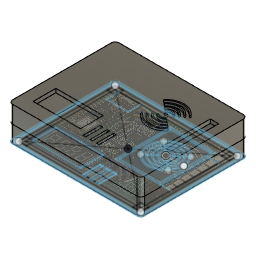
RFIDBox v2 (Autodesk Fusion 360 design; units mm, degrees)
Autodesk Fusion 360 part; units mm, degrees
note: some values were not read from the file. Chosen so that the rebuilt part matches the saved one: which bodies a step acts on; which face or edge a step refers to. Set by a fixed rule: which sketch regions a step uses.
sketch "Sketch1" plane through (0, 0, 0) normal (0, 0, 1) x (1, 0, 0)
  line L0 (47.5, -37.5) -> (-47.5, -37.5)
  line L1 (-47.5, -37.5) -> (-47.5, 37.5)
  line L2 (-47.5, 37.5) -> (47.5, 37.5)
  line L3 (47.5, 37.5) -> (47.5, -37.5)
  line L4 (47.5, -37.5) -> (-47.5, 37.5) construction
  line L5 (-47.5, -37.5) -> (47.5, 37.5) construction
  line L6 (45, -35) -> (-45, -35)
  line L7 (-45, -35) -> (-45, 35)
  line L8 (-45, 35) -> (45, 35)
  line L9 (45, 35) -> (45, -35)
  line L10 (45, -35) -> (-45, 35) construction
  line L11 (-45, -35) -> (45, 35) construction
  line L12 (-42.4055, -13.8661) -> (-5.5569, -13.8661)
  line L13 (-5.5569, -13.8661) -> (-5.5569, -31.5415)
  line L14 (-5.5569, -31.5415) -> (-42.4055, -31.5415)
  line L15 (-42.4055, -31.5415) -> (-42.4055, -13.8661)
  line L16 (38.4816, 25.6787) -> (45, 25.6787)
  line L17 (45, 25.6787) -> (45, -11.6193)
  line L18 (45, -11.6193) -> (38.4816, -11.6193)
  line L19 (38.4816, -11.6193) -> (38.4816, 25.6787)
  line L20 (2.0824, 31.0711) -> (36.6841, 31.0711)
  line L21 (36.6841, 31.0711) -> (36.6841, -11.6193)
  line L22 (36.6841, -11.6193) -> (2.0824, -11.6193)
  line L23 (2.0824, -11.6193) -> (2.0824, 31.0711)
  line L24 (-41.6565, 35) -> (-25, 35)
  line L25 (-25, 35) -> (-25, 25)
  line L26 (-25, 25) -> (-41.6565, 25)
  line L27 (-41.6565, 25) -> (-41.6565, 35)
  line L28 (0, -21.6553) -> (12.418, -21.6553)
  line L29 (12.418, -21.6553) -> (12.418, -35)
  line L30 (12.418, -35) -> (0, -35)
  line L31 (0, -35) -> (0, -21.6553)
  line L32 (-48.5, 41.5) -> (48.5, 41.5)
  line L33 (51.5, 38.5) -> (51.5, -38.5)
  line L34 (48.5, -41.5) -> (-48.5, -41.5)
  line L35 (-51.5, -38.5) -> (-51.5, 38.5)
  line L36 (-47.5, 39.5) -> (47.5, 39.5)
  line L37 (49.5, 37.5) -> (49.5, -37.5)
  line L38 (47.5, -39.5) -> (-47.5, -39.5)
  line L39 (-49.5, -37.5) -> (-49.5, 37.5)
  line L40 (-47.5, 37.5) -> (-41.5, 37.5)
  line L41 (-41.5, 37.5) -> (-41.5, 31.5)
  line L42 (-41.5, 31.5) -> (-47.5, 31.5)
  line L43 (-47.5, 31.5) -> (-47.5, 37.5)
  line L44 (-47.5, -37.5) -> (-41.5, -37.5)
  line L45 (-41.5, -37.5) -> (-41.5, -31.5)
  line L46 (-41.5, -31.5) -> (-47.5, -31.5)
  line L47 (-47.5, -31.5) -> (-47.5, -37.5)
  line L48 (47.5, 37.5) -> (41.5, 37.5)
  line L49 (41.5, 37.5) -> (41.5, 31.5)
  line L50 (41.5, 31.5) -> (47.5, 31.5)
  line L51 (47.5, 31.5) -> (47.5, 37.5)
  line L52 (47.5, -37.5) -> (41.5, -37.5)
  line L53 (41.5, -37.5) -> (41.5, -31.5)
  line L54 (41.5, -31.5) -> (47.5, -31.5)
  line L55 (47.5, -31.5) -> (47.5, -37.5)
  arc A0 (-48.5, 41.5) -> (-51.5, 38.5) centre (-48.5, 38.5) ccw
  arc A1 (51.5, 38.5) -> (48.5, 41.5) centre (48.5, 38.5) ccw
  arc A2 (48.5, -41.5) -> (51.5, -38.5) centre (48.5, -38.5) ccw
  arc A3 (-51.5, -38.5) -> (-48.5, -41.5) centre (-48.5, -38.5) ccw
  arc A4 (-47.5, 39.5) -> (-49.5, 37.5) centre (-47.5, 37.5) ccw
  arc A5 (-49.5, -37.5) -> (-47.5, -39.5) centre (-47.5, -37.5) ccw
  arc A6 (47.5, -39.5) -> (49.5, -37.5) centre (47.5, -37.5) ccw
  arc A7 (49.5, 37.5) -> (47.5, 39.5) centre (47.5, 37.5) ccw
  line L56 (-50, -37.5) -> (-50, 37.5)
  arc A8 (-47.5, 40) -> (-50, 37.5) centre (-47.5, 37.5) ccw
  line L57 (-47.5, 40) -> (47.5, 40)
  arc A9 (50, 37.5) -> (47.5, 40) centre (47.5, 37.5) ccw
  line L58 (50, 37.5) -> (50, -37.5)
  arc A10 (47.5, -40) -> (50, -37.5) centre (47.5, -37.5) ccw
  line L59 (47.5, -40) -> (-47.5, -40)
  arc A11 (-50, -37.5) -> (-47.5, -40) centre (-47.5, -37.5) ccw
  line L60 (0, -21.6553) -> (2, -21.6553)
  line L61 (2, -21.6553) -> (2, -35)
  line L62 (2, -35) -> (0, -35)
  line L63 (0, -35) -> (0, -21.6553)
  line L64 (12.418, -21.6553) -> (10.418, -21.6553)
  line L65 (10.418, -21.6553) -> (10.418, -35)
  line L66 (10.418, -35) -> (12.418, -35)
  line L67 (12.418, -35) -> (12.418, -21.6553)
  line L68 (5.4095, -21.6553) -> (7.4095, -21.6553)
  line L69 (7.4095, -21.6553) -> (7.4095, -35)
  line L70 (7.4095, -35) -> (5.4095, -35)
  line L71 (5.4095, -35) -> (5.4095, -21.6553)
  line L72 (3.5824, 29.5711) -> (35.1841, 29.5711)
  line L73 (35.1841, 29.5711) -> (35.1841, -10.1193)
  line L74 (35.1841, -10.1193) -> (3.5824, -10.1193)
  line L75 (3.5824, -10.1193) -> (3.5824, 29.5711)
  circle A12 centre (19.3833, 10.1139) radius 1
  circle A13 centre (19.3833, 10.1139) radius 4
  circle A14 centre (19.3833, 10.1139) radius 5
  circle A15 centre (19.3833, 10.1139) radius 7
  circle A16 centre (19.3833, 10.1139) radius 8
  circle A17 centre (19.3833, 10.1139) radius 10
  circle A18 centre (19.3833, 10.1139) radius 11
  circle A19 centre (19.3833, 10.1139) radius 13
  circle A20 centre (19.3833, 10.1139) radius 14
  line L76 (19.3833, 10.1139) -> (8.6587, 19.1129)
  line L77 (19.3833, 10.1139) -> (33.3833, 10.1139) construction
  line L78 (19.3833, 10.1139) -> (30.1079, 1.1149)
  line L79 (19.3833, 10.1139) -> (33.3833, 10.1139) construction
  line L80 (19.3833, 10.1139) -> (30.1079, 19.1129)
  line L81 (19.3833, 10.1139) -> (33.3833, 10.1139) construction
  line L82 (19.3833, 10.1139) -> (8.6587, 1.1149)
  line L83 (19.3833, 10.1139) -> (33.3833, 10.1139) construction
  dimension "d1" = 95
  dimension "d2" = 75
  dimension "d3" = 90
  dimension "d4" = 70
  dimension "d9" = 6
  dimension "d10" = 6
  dimension "d11" = 6
  dimension "d12" = 6
  dimension "d13" = 6
  dimension "d14" = 6
  dimension "d15" = 6
  dimension "d16" = 6
  dimension "d25" = 3
  dimension "d26" = 3
  dimension "d27" = 3
  dimension "d28" = 3
  dimension "d29" = 2
  dimension "d30" = 2
  dimension "d31" = 2
  dimension "d32" = 2
  dimension "d33" = -0.5
  dimension "d44" = 2
  dimension "d45" = 2
  dimension "d46" = 2
  dimension "d51" = 1.5
  dimension "d52" = 2
  dimension "d53" = 8
  dimension "d54" = 10
  dimension "d55" = 14
  dimension "d56" = 16
  dimension "d57" = 20
  dimension "d58" = 22
  dimension "d59" = 26
  dimension "d60" = 28
  dimension "d61" = 140
  dimension "d62" = 40
  dimension "d63" = 40
  dimension "d64" = 140
  constraint horizontal L0
  constraint perpendicular L0 L1
  constraint parallel L0 L2
  constraint parallel L1 L3
  constraint coincident L4 origin
  constraint coincident L5 origin
  constraint horizontal L6
  constraint perpendicular L6 L7
  constraint parallel L6 L8
  constraint parallel L7 L9
  constraint coincident L10 origin
  constraint coincident L11 origin
  constraint horizontal L12
  constraint vertical L13
  constraint horizontal L14
  constraint vertical L15
  constraint horizontal L16
  constraint vertical L17
  constraint horizontal L18
  constraint vertical L19
  constraint coincident L9 L17.end
  constraint horizontal L20
  constraint vertical L21
  constraint horizontal L22
  constraint vertical L23
  constraint horizontal L24
  constraint vertical L25
  constraint horizontal L26
  constraint vertical L27
  constraint coincident L8 L24.start
  constraint horizontal L28
  constraint vertical L29
  constraint horizontal L30
  constraint vertical L31
  constraint coincident L6 L29.end
  constraint horizontal L40
  constraint vertical L41
  constraint horizontal L42
  constraint vertical L43
  constraint horizontal L44
  constraint vertical L45
  constraint horizontal L46
  constraint vertical L47
  constraint horizontal L48
  constraint vertical L49
  constraint horizontal L50
  constraint vertical L51
  constraint horizontal L52
  constraint vertical L53
  constraint horizontal L54
  constraint vertical L55
  constraint parallel L2 L32
  constraint parallel L3 L33
  constraint parallel L0 L34
  constraint parallel L1 L35
  constraint tangent L32 A0
  constraint tangent L35 A0
  constraint tangent L32 A1
  constraint tangent L33 A1
  constraint tangent L33 A2
  constraint tangent L34 A2
  constraint tangent L34 A3
  constraint tangent L35 A3
  constraint parallel L2 L36
  constraint parallel L3 L37
  constraint parallel L0 L38
  constraint parallel L1 L39
  constraint tangent L36 A4
  constraint tangent L39 A4
  constraint tangent L38 A5
  constraint tangent L39 A5
  constraint tangent L37 A6
  constraint tangent L38 A6
  constraint tangent L36 A7
  constraint tangent L37 A7
  constraint horizontal L60
  constraint vertical L61
  constraint horizontal L62
  constraint vertical L63
  constraint horizontal L64
  constraint vertical L65
  constraint horizontal L66
  constraint vertical L67
  constraint horizontal L68
  constraint vertical L69
  constraint horizontal L70
  constraint vertical L71
  constraint coincident L28 L68.start
  constraint concentric A12 A13
  constraint concentric A12 A14
  constraint concentric A14 A15
  constraint concentric A15 A16
  constraint concentric A12 A17
  constraint concentric A12 A18
  constraint concentric A18 A19
  constraint concentric A18 A20
  constraint horizontal L77
  constraint coincident A12.centre A13.centre
  constraint horizontal L79
  constraint horizontal L81
  constraint horizontal L83
  measures "d1" distance of L1.end L2.end
  measures "d2" distance of L0.end L1.end
  measures "d3" distance of L7.end L8.end
  measures "d4" distance of L6.end L7.end
  measures "d9" distance of L1.end L40.end
  measures "d10" distance of L1.end L42.end
  measures "d11" distance of L0.end L44.end
  measures "d12" distance of L0.end L46.end
  measures "d13" distance of L2.end L48.end
  measures "d14" distance of L2.end L50.end
  measures "d15" distance of L0.start L52.end
  measures "d16" distance of L0.start L54.end
  measures "d25" radius of A0
  measures "d26" radius of A1
  measures "d27" radius of A2
  measures "d28" radius of A3
  measures "d29" radius of A4
  measures "d30" radius of A5
  measures "d31" radius of A6
  measures "d32" radius of A7
  measures "d44" distance of L28.start L60.end
  measures "d45" distance of L28.end L64.end
  measures "d46" distance of L68.start L68.end
  measures "d52" diameter of A12
  measures "d53" diameter of A13
  measures "d54" diameter of A14
  measures "d55" diameter of A15
  measures "d56" diameter of A16
  measures "d57" diameter of A17
  measures "d58" diameter of A18
  measures "d59" diameter of A19
  measures "d60" diameter of A20
  measures "d61" angle of L76 L77
  measures "d62" angle of L78 L79
  measures "d63" angle of L80 L81
  measures "d64" angle of L82 L83
extrude "Extrude13" add sketch "Sketch1" along normal blind 1.5 contours A12 L78 L80 | A12 L76 L80 | A12 L78 L82 | A12 L76 L82 | A13 A14 L76 L80 | A13 A14 L78 L82 | A15 A16 L76 L80 | A15 A16 L78 L82 | A17 A18 L76 L80 | A17 A18 L78 L82 | A19 A20 L76 L80 | A19 A20 L78 L82 makes body 1 at (27.4572, 2.6432, 1) makes body 2 at (13.5113, 15.5471, 1) makes body 3 at (11.3093, 17.5846, 1) makes body 4 at (16.7201, 2.5702, 1) makes body 5 at (18.7048, -3.8697, 1) makes body 6 at (19.8673, 15.0904, 1) makes body 7 at (12.266, 22.1698, 0.5) makes body 8 at (20.5835, 5.2601, 1) makes body 9 at (20.3783, 10.0143, 0.5)
extrude "Extrude6" add sketch "Sketch1" against normal blind 3 separate body contours L0 L3 L6 L9 L52 L53 L54 L55 | L0 L6 L30 L45 L53 L62 L66 L70 | L3 L9 L17 L50 L54 | L0 L1 L6 L7 L44 L45 L46 L47 | L6 L9 L53 L54 | L6 L7 L8 L9 L12 L13 L14 L15 L16 L18 L19 L25 L26 L27 L28 L29 L31 L42 L45 L46 L49 L50 L53 L54 L60 L63 L64 L67 L68 | L2 L3 L8 L9 L48 L49 L50 L51 | L6 L7 L14 L15 L45 L46 | L6 L28 L29 L30 L64 L65 L66 L67 | L8 L9 L49 L50 | L9 L16 L17 L18 L19 | L1 L7 L42 L46 | L6 L28 L30 L31 L60 L61 L62 L63 | L12 L13 L14 L15 L45 L46 | L14 L15 L45 L46 | L6 L28 L30 L65 L69 | L2 L8 L24 L41 L49 | L1 L2 L7 L8 L24 L40 L41 L42 L43 | L6 L28 L30 L61 L71 | L6 L28 L30 L68 L69 L70 L71 | L7 L8 L27 L42 | L8 L24 L27 L41 L42 | L8 L24 L25 L26 L27 L41 L42 | L20 L21 L22 L23 | L32 L33 L34 L35 A0 A1 A2 A3 | L36 L37 L38 L39 A4 A5 A6 A7 | L56 A8 L57 A9 L58 A10 L59 A11 | L72 L73 L74 L75 | A12 L78 L80 | A12 A13 L78 L80 | A12 L76 L80 | A12 A13 L76 L80 | A12 A13 L78 L82 | A12 L78 L82 | A12 L76 L82 | A12 A13 L76 L82 | A13 A14 L78 L80 | A13 A14 L76 L80 | A13 A14 L78 L82 | A13 A14 L76 L82 | A14 A15 L78 L80 | A14 A15 L76 L80 | A14 A15 L78 L82 | A14 A15 L76 L82 | A15 A16 L78 L80 | A15 A16 L76 L80 | A15 A16 L78 L82 | A15 A16 L76 L82 | A16 A17 L78 L80 | A16 A17 L76 L80 | A16 A17 L78 L82 | A16 A17 L76 L82 | A17 A18 L78 L80 | A17 A18 L76 L80 | A17 A18 L78 L82 | A17 A18 L76 L82 | A18 A19 L78 L80 | A18 A19 L76 L80 | A18 A19 L78 L82 | A18 A19 L76 L82 | A19 A20 L78 L80 | A19 A20 L76 L80 | A19 A20 L78 L82 | A19 A20 L76 L82 makes body 10
extrude "Extrude2" add sketch "Sketch1" along normal blind 6 separate body contours L0 L3 L6 L9 L52 L53 L54 L55 | L0 L1 L6 L7 L44 L45 L46 L47 | L6 L9 L53 L54 | L2 L3 L8 L9 L48 L49 L50 L51 | L6 L7 L14 L15 L45 L46 | L8 L9 L49 L50 | L14 L15 L45 L46 | L1 L2 L7 L8 L24 L40 L41 L42 L43 | L7 L8 L27 L42 | L8 L24 L27 L41 L42 makes body 11 at (43.5, 31.5, 4) makes body 12 at (45.5, -37.5, 4) makes body 13 at (-43.5, 31.5, 4) makes body 14 at (-43.5, -31.5, 4)
extrude "Extrude1" add sketch "Sketch1" along normal blind 3 separate body contours L0 L3 L6 L9 L52 L53 L54 L55 | L0 L6 L30 L45 L53 L62 L66 L70 | L3 L9 L17 L50 L54 | L0 L1 L6 L7 L44 L45 L46 L47 | L6 L9 L53 L54 | L6 L7 L8 L9 L12 L13 L14 L15 L16 L18 L19 L25 L26 L27 L28 L29 L31 L42 L45 L46 L49 L50 L53 L54 L60 L63 L64 L67 L68 | L2 L3 L8 L9 L48 L49 L50 L51 | L6 L7 L14 L15 L45 L46 | L6 L28 L29 L30 L64 L65 L66 L67 | L8 L9 L49 L50 | L9 L16 L17 L18 L19 | L1 L7 L42 L46 | L6 L28 L30 L31 L60 L61 L62 L63 | L12 L13 L14 L15 L45 L46 | L14 L15 L45 L46 | L6 L28 L30 L65 L69 | L2 L8 L24 L41 L49 | L1 L2 L7 L8 L24 L40 L41 L42 L43 | L6 L28 L30 L61 L71 | L6 L28 L30 L68 L69 L70 L71 | L7 L8 L27 L42 | L8 L24 L27 L41 L42 | L8 L24 L25 L26 L27 L41 L42 | L20 L21 L22 L23 | L32 L33 L34 L35 A0 A1 A2 A3 | L36 L37 L38 L39 A4 A5 A6 A7 | L56 A8 L57 A9 L58 A10 L59 A11 | L72 L73 L74 L75 | A12 L78 L80 | A12 A13 L78 L80 | A12 L76 L80 | A12 A13 L76 L80 | A12 A13 L78 L82 | A12 L78 L82 | A12 L76 L82 | A12 A13 L76 L82 | A13 A14 L78 L80 | A13 A14 L76 L80 | A13 A14 L78 L82 | A13 A14 L76 L82 | A14 A15 L78 L80 | A14 A15 L76 L80 | A14 A15 L78 L82 | A14 A15 L76 L82 | A15 A16 L78 L80 | A15 A16 L76 L80 | A15 A16 L78 L82 | A15 A16 L76 L82 | A16 A17 L78 L80 | A16 A17 L76 L80 | A16 A17 L78 L82 | A16 A17 L76 L82 | A17 A18 L78 L80 | A17 A18 L76 L80 | A17 A18 L78 L82 | A17 A18 L76 L82 | A18 A19 L78 L80 | A18 A19 L76 L80 | A18 A19 L78 L82 | A18 A19 L76 L82 | A19 A20 L78 L80 | A19 A20 L76 L80 | A19 A20 L78 L82 | A19 A20 L76 L82 makes body 15
extrude "Extrude3" add sketch "Sketch1" along normal blind 26 contours L36 L37 L38 L39 A4 A5 A6 A7 bodies 11 12 13 14
combine "Combine1" operation add target body 15 tool bodies 11
extrude "Extrude4" add 1 faces at (-15.8333, 40.8333, 3) along direction (0, 0, 1) blind 10 on bodies 15 bodies 15
extrude "Extrude5" add 1 faces at (-15.8333, 40.8333, 13) along direction (0, 0, 1) blind 3 on bodies 15 bodies 15
extrude "Extrude7" add sketch "Sketch1" against normal blind 13.5 contours L32 L33 L34 L35 A0 A1 A2 A3 bodies 10
extrude "Extrude8" cut 1 faces at (-15.8333, 40.8333, 16) along direction (0, 0, -1) blind 3 on bodies 15 bodies 15
extrude "Extrude9" cut 1 faces at (-15.8333, -38.1667, 26) along direction (0, 0, -1) blind 3 on bodies 15 bodies 15
extrude "Extrude10" cut sketch "Sketch1" against normal blind 20 contours L12 L13 L14 L15 L45 L46 bodies 10
extrude "Extrude11" cut sketch "Sketch1" against normal blind 10 contours L6 L28 L29 L30 L64 L65 L66 L67 | L6 L28 L30 L31 L60 L61 L62 L63 | L6 L28 L30 L68 L69 L70 L71 bodies 10
extrude "Extrude12" cut sketch "Sketch1" against normal blind 5 contours L9 L16 L17 L18 L19 bodies 10
combine "Combine2" operation add target body 10 tool bodies 1 2 3 4 5 6 7 8 9
move_body "Move1" bodies 10 to x (1, 0, 0) y (0, 1, 0) z (0, 0, 1) at (0, 0, 26.5)
sketch "Sketch2" plane through (0, 41.5, 0) normal (0, 1, 0) x (-1, 0, 0)
  line L0 (48.5, 26.5) -> (-48.5, 26.5)
  line L1 (-48.5, 26.5) -> (-48.5, 13)
  line L2 (-48.5, 13) -> (48.5, 13)
  line L3 (48.5, 13) -> (48.5, 26.5)
  line L4 (43, 23) -> (23, 23)
  line L5 (23, 23) -> (23, 13)
  line L6 (23, 13) -> (43, 13)
  line L7 (43, 13) -> (43, 23)
  dimension "d67" = 20
  constraint horizontal L4
  constraint vertical L5
  constraint horizontal L6
  constraint vertical L7
  measures "d67" distance of L4.start L4.end
extrude "Extrude14" cut sketch "Sketch2" against normal blind 10 contours L2 L4 L5 L6 L7 bodies 10 15
